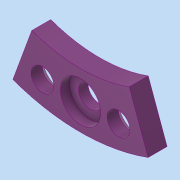
# Autodesk Inventor part: pushSwitchBushingHolder
Saved by Autodesk Inventor 2017 (Build 210142000, 142)
## iProperties
Created: 2016-12-03
Part Number: pushSwitchBushingHolder
Material: ABS Plastic
Document SubType Name: Modeling
Designer: techn
Density: 1.06 g/cm^3
Appearance: Smooth - Purple
Author: techn
Autodesk Inventor part; units mm, degrees
ref_plane "YZ Plane" through (0, 0, 0) normal (1, 0, 0) x (0, 1, 0)
ref_plane "XZ Plane" through (0, 0, 0) normal (0, 1, 0) x (-1, 0, 0)
ref_plane "XY Plane" through (0, 0, 0) normal (0, 0, 1) x (1, 0, 0)
sketch "Sketch1" plane through (0, 0, 0) normal (0, 0, 1) x (1, 0, 0)
  circle A0 centre (0, 0) radius 1.905
  circle A1 centre (0, 0) radius 3.3655
  line L0 (0, 0) -> (0, 28.575)
  line L1 (0, 0) -> (28.575, 0) construction
  circle A2 centre (0, 28.575) radius 33.02
  line L2 (0, 0) -> (6.35, 0)
  line L3 (6.35, 0) -> (-6.35, 0)
  circle A3 centre (-6.35, 0) radius 1.905
  circle A4 centre (6.35, 0) radius 1.905
  line L4 (0, 28.575) -> (11.2935, -2.4537)
  line L5 (0, 28.575) -> (33.02, 28.575) construction
  line L6 (0, 28.575) -> (-11.2935, -2.4537)
  circle A5 centre (0, 28.575) radius 23.8125
  dimension "d0" = 3.81
  dimension "d1" = 6.731
  dimension "d3" = 28.575
  dimension "d4" = 90
  dimension "d5" = 66.04
  dimension "d6" = 6.35
  dimension "d7" = 12.7
  dimension "d8" = 3.81
  dimension "d9" = 3.81
  dimension "d10" = 70
  dimension "d11" = 47.625
  constraints: 14 end point, 7 coincident, 6 centre point, 2 equal length, 2 horizontal, 2 point on circle, 2 point on line, 1 vertical
  measures "d0" diameter of A0
  measures "d1" diameter of A1
  measures "d3" distance of L0.start L0.end
  measures "d4" angle of L1 L0
  measures "d5" diameter of A2
  measures "d6" distance of L0.start L2.end
  measures "d7" distance of L2.end L3.end
  measures "d8" diameter of A3
  measures "d9" diameter of A4
  measures "d10" angle of L4 L5
  measures "d11" diameter of A5
extrude "Extrusion1" add sketch "Sketch1" against normal blind 3.175 contours L2 A1 L3 A0 | A0 L0 A1 L2 | A0 L3 A1 L0 | A5 L6 L0 | A5 L4 A2 L6 | L0 L4 A5 picked at (9.1582, 1.5434)
extrude "Extrusion2" cut sketch "Sketch1" against normal blind 1.5875 contours L2 A1 L3 A0 | A0 L0 A1 L2 | A0 L3 A1 L0
extrude "Extrusion3" cut sketch "Sketch1" against normal through all contours A5 L6 L0 | L0 L4 A5 | L6 A5 L4
chamfer "Chamfer1" distance 1.27 angle 45 2 edges at (4.445, 0, -3.175) (-8.255, 0, -3.175)
equation "\"d9\" = d8"
body "Solid1"
